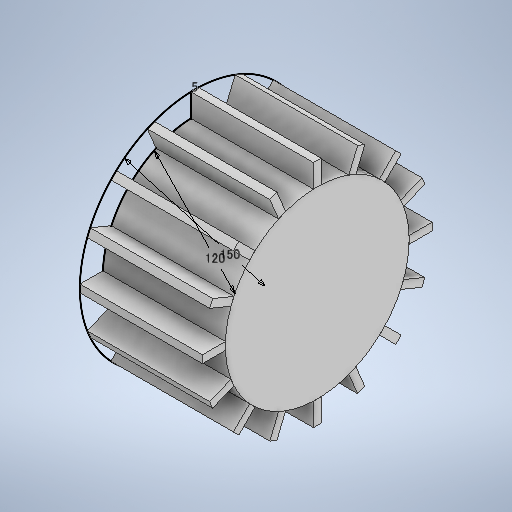
# Autodesk Inventor part: wheel
Saved by Autodesk Inventor 2027.1 (Build 311270010, 270A)
## iProperties
Created: 2025-08-18
Part Number: wheel
Material: 一般
Document SubType Name: Modeling
Designer: moonshot
Density: 1 g/cm^3
Appearance: 既定
Author: moonshot
Autodesk Inventor part; units mm, degrees
ref_plane "YZ Plane" through (0, 0, 0) normal (1, 0, 0) x (0, 1, 0)
ref_plane "XZ Plane" through (0, 0, 0) normal (0, 1, 0) x (-1, 0, 0)
ref_plane "XY Plane" through (0, 0, 0) normal (0, 0, 1) x (1, 0, 0)
sketch "スケッチ1" plane through (0, 0, 0) normal (1, 0, 0) x (0, 1, 0)
  circle A0 centre (0, 0) radius 75
  circle A1 centre (0, 0) radius 60
  line L0 (45, 2.5) -> (75, 2.5)
  line L1 (75, 2.5) -> (75, -2.5)
  line L2 (75, -2.5) -> (45, -2.5)
  line L3 (45, -2.5) -> (45, 2.5)
  line L4 (45, 2.5) -> (75, -2.5) construction
  line L5 (75, 2.5) -> (45, -2.5) construction
  line L6 (75, 0) -> (0, 0)
  point P0 (60, 0)
  point P1 (59.9479, -2.5)
  point P2 (74.9583, -2.5)
  point P3 (74.9583, 2.5)
  point P4 (59.9479, 2.5)
  dimension "d0" = 150
  dimension "d1" = 120
  dimension "d2" = 5
  constraints: 14 end point, 2 coincident, 2 horizontal, 2 midpoint, 2 parallel, 1 perpendicular, 1 symmetric about line, 1 vertical, 6 other
  measures "d2" distance of L0.end L1.end
extrude "押し出し1" add sketch "スケッチ1" along normal blind 80 contours L6 L3 L0 A1 | A1 L2 L3 L6 | L0 L3 L2 A1
extrude "押し出し2" add sketch "スケッチ1" along normal blind 80 separate body contours L6 A1 L0 A0 | A0 L2 A1 L6
pattern_circular "円形状パターン1" count 16 over 360 about axis through (-10, 0, 0) along (1, 0, 0) of "押し出し2" bodies 2
